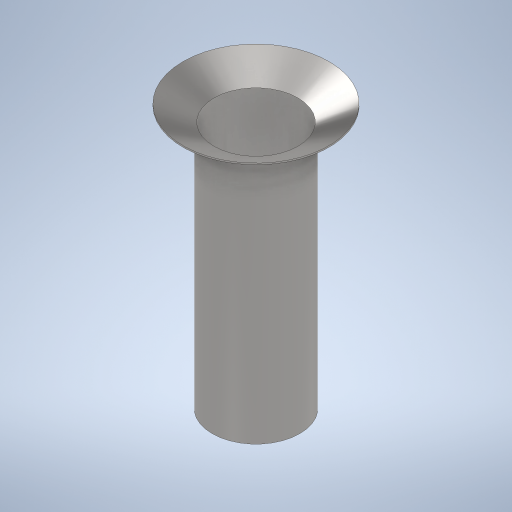
# Autodesk Inventor part: Trash bin casing X1
Saved by Autodesk Inventor 2023 (Build 270158000, 158)
## iProperties
Created: 2022-11-23
Part Number: Trash bin casing X1
Material: Stainless Steel
Document SubType Name: Modeling
Designer: surat
Density: 8 g/cm^3
Appearance: Semi-Polished
Author: surat
Autodesk Inventor part; units mm, degrees
ref_plane "YZ Plane" through (0, 0, 0) normal (1, 0, 0) x (0, 1, 0)
ref_plane "XZ Plane" through (0, 0, 0) normal (0, 1, 0) x (-1, 0, 0)
ref_plane "XY Plane" through (0, 0, 0) normal (0, 0, 1) x (1, 0, 0)
sketch "Sketch1" plane through (0, 0, 0) normal (0, 1, 0) x (-1, 0, 0)
  circle A0 centre (0, 0) radius 152.4
  circle A1 centre (0, 0) radius 146.05
  dimension "d0" = 304.8
  dimension "d1" = 6.35
  constraints: 2 centre point, 1 coincident
  measures "d0" diameter of A0
  measures "d1" radial gap between concentric circles of A0 A1
extrude "Extrusion1" add sketch "Sketch1" along normal blind 863.6
extrude "Extrusion2" add sketch "Sketch1" along normal blind 6.35 contours A1
sketch "Sketch2" plane through (0, 6.35, 0) normal (0, 1, 0) x (1, 0, 0)
  line L0 (-219.9994, 0) -> (351.4578, 0)
  point P0 (0, 0)
  constraints: 2 end point, 1 horizontal
ref_plane "Work Plane1" through (-219.9994, 6.35, 0) normal (0, 0, 1) x (1, 0, 0)
sketch "Sketch3" plane through (-219.9994, 6.35, 0) normal (0, 0, 1) x (1, 0, 0)
  line L0 (372.3994, 857.25) -> (67.5994, 857.25) projected
  line L1 (67.5994, 857.25) -> (67.5994, 913.13)
  line L2 (67.5994, 913.13) -> (-34.0006, 913.13)
  line L3 (-34.0006, 913.13) -> (-34.0006, 908.05)
  line L4 (-34.0006, 908.05) -> (67.5994, 857.25)
  line L5 (73.9494, 857.25) -> (366.0494, 857.25) projected
  line L6 (73.9494, 857.25) -> (-34.0006, 913.13)
  line L7 (219.9994, 947.7824) -> (219.9994, 874.9501)
  point P0 (219.9994, -6.35)
  dimension "d6" = 55.88
  dimension "d7" = 101.6
  dimension "d8" = 5.08
  constraints: 12 end point, 3 vertical, 1 horizontal
  measures "d6" distance of L0.end L1.end
  measures "d7" distance of L1.end L2.end
  measures "d8" distance of L2.end L3.end
revolve "Revolution1" add sketch "Sketch3" angle 360 about axis through (0, 954.1324, 0) along (0, -1, 0) contours L0 L1 L6 | L4 L3 L6 L1
body "Solid1"
